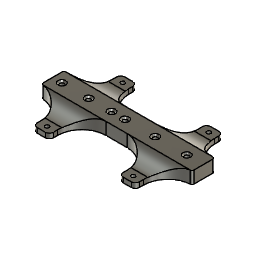
base (Autodesk Fusion 360 design; units mm, degrees)
Autodesk Fusion 360 part; units mm, degrees
sketch "Sketch1" plane through (0, 0, 0) normal (0, 0, 1) x (1, 0, 0)
  line L0 (0, 0) -> (186, 0)
  line L1 (186, 0) -> (186, 28)
  line L2 (186, 28) -> (0, 28)
  line L3 (0, 28) -> (0, 0)
  line L4 (0, 14) -> (186, 14) construction
  circle A0 centre (11.5, 14) radius 2.75
  circle A1 centre (44.5, 14) radius 2.75
  circle A2 centre (72.6667, 14) radius 2.75
  circle A3 centre (89.3333, 14) radius 2.75
  circle A4 centre (126.5, 14) radius 2.75
  circle A5 centre (165.5, 14) radius 2.75
  line L5 (13.8094, 10) -> (16.1188, 14)
  line L6 (16.1188, 14) -> (13.8094, 18)
  line L7 (13.8094, 18) -> (9.1906, 18)
  line L8 (9.1906, 18) -> (6.8812, 14)
  line L9 (6.8812, 14) -> (9.1906, 10)
  line L10 (9.1906, 10) -> (13.8094, 10)
  line L11 (46.8094, 10) -> (49.1188, 14)
  line L12 (49.1188, 14) -> (46.8094, 18)
  line L13 (46.8094, 18) -> (42.1906, 18)
  line L14 (42.1906, 18) -> (39.8812, 14)
  line L15 (39.8812, 14) -> (42.1906, 10)
  line L16 (42.1906, 10) -> (46.8094, 10)
  line L17 (74.9761, 10) -> (77.2855, 14)
  line L18 (77.2855, 14) -> (74.9761, 18)
  line L19 (74.9761, 18) -> (70.3573, 18)
  line L20 (70.3573, 18) -> (68.0479, 14)
  line L21 (68.0479, 14) -> (70.3573, 10)
  line L22 (70.3573, 10) -> (74.9761, 10)
  line L23 (91.6427, 10) -> (93.9521, 14)
  line L24 (93.9521, 14) -> (91.6427, 18)
  line L25 (91.6427, 18) -> (87.0239, 18)
  line L26 (87.0239, 18) -> (84.7145, 14)
  line L27 (84.7145, 14) -> (87.0239, 10)
  line L28 (87.0239, 10) -> (91.6427, 10)
  line L29 (128.8094, 10) -> (131.1188, 14)
  line L30 (131.1188, 14) -> (128.8094, 18)
  line L31 (128.8094, 18) -> (124.1906, 18)
  line L32 (124.1906, 18) -> (121.8812, 14)
  line L33 (121.8812, 14) -> (124.1906, 10)
  line L34 (124.1906, 10) -> (128.8094, 10)
  line L35 (167.8094, 10) -> (170.1188, 14)
  line L36 (170.1188, 14) -> (167.8094, 18)
  line L37 (167.8094, 18) -> (163.1906, 18)
  line L38 (163.1906, 18) -> (160.8812, 14)
  line L39 (160.8812, 14) -> (163.1906, 10)
  line L40 (163.1906, 10) -> (167.8094, 10)
  point P0 (11.5, 14)
  point P1 (44.5, 14)
  point P2 (72.6667, 14)
  point P3 (89.3333, 14)
  point P4 (126.5, 14)
  point P5 (165.5, 14)
  dimension "d1" = 186
  dimension "d2" = 28
  dimension "d3" = 5.5
  dimension "d4" = 11.5
  dimension "d5" = 5.5
  dimension "d6" = 44.5
  dimension "d7" = 5.5
  dimension "d8" = 5.5
  dimension "d9" = 5.5
  dimension "d10" = 5.5
  dimension "d11" = 72.6667
  dimension "d12" = 89.3333
  dimension "d13" = 20.5
  dimension "d14" = 126.5
  dimension "d18" = 4
  dimension "d19" = 4
  dimension "d20" = 4
  dimension "d21" = 4
  dimension "d22" = 4
  dimension "d23" = 4
  constraint horizontal L0
  constraint vertical L1
  constraint horizontal L2
  constraint vertical L3
  constraint coincident L0.start L3.end
  constraint midpoint L3 L4.start
  constraint midpoint L1 L4.end
  constraint coincident L4 P0
  constraint coincident L4 P1
  constraint coincident L4 P2
  constraint coincident L4 P3
  constraint coincident L4 P4
  constraint coincident L4 P5
  constraint coincident P0 A0.centre
  constraint coincident P1 A1.centre
  constraint coincident P2 A2.centre
  constraint coincident P3 A3.centre
  constraint coincident P4 A4.centre
  constraint coincident P5 A5.centre
  measures "d1" distance of L0.start L0.end
  measures "d2" distance of L0.start L2.end
  measures "d3" diameter of A0
  measures "d4" distance of L4.start P0
  measures "d5" diameter of A1
  measures "d6" distance of L3 P1
  measures "d7" diameter of A2
  measures "d8" diameter of A3
  measures "d9" diameter of A4
  measures "d10" diameter of A5
  measures "d11" distance of L3 P2
  measures "d12" distance of L3 P3 L0.start
  measures "d13" distance of L1 P5
  measures "d14" distance of L3 P4
  measures "d18" distance of P0 L10
  measures "d19" distance of P1 L16
  measures "d20" distance of P2 L22
  measures "d21" distance of P3 L28
  measures "d22" distance of P4 L34
  measures "d23" distance of P5 L40
extrude "Extrude1" add sketch "Sketch1" along normal blind 15 contours L0 L1 L2 L3 | L5 L6 L7 L8 L9 L10 | L11 L12 L13 L14 L15 L16 | L17 L18 L19 L20 L21 L22 | L23 L24 L25 L26 L27 L28 | L29 L30 L31 L32 L33 L34 | L35 L36 L37 L38 L39 L40
chamfer "Chamfer1" distance 2 angle 45 6 edges at (8.9361, 14.9944, 15) (41.9361, 14.9944, 15) (70.1028, 14.9944, 15) (86.7694, 14.9944, 15) (123.9361, 14.9944, 15) (162.9361, 14.9944, 15)
extrude "Extrude2" cut sketch "Sketch1" along normal blind 4 contours L5 L6 L7 L8 L9 L10 | L11 L12 L13 L14 L15 L16 | L17 L18 L19 L20 L21 L22 | L23 L24 L25 L26 L27 L28 | L29 L30 L31 L32 L33 L34 | L35 L36 L37 L38 L39 L40
sketch "Sketch2" plane through (0, 0, 0) normal (-1, 0, 0) x (0, -1, 0)
  line L0 (-28, 0) -> (0, 0)
  line L1 (0, 0) -> (0, 15)
  line L2 (0, 15) -> (-28, 15)
  line L3 (-28, 15) -> (-28, 0)
  line L4 (0, 0) -> (40, 0)
  line L5 (40, 0) -> (40, 6)
  line L6 (40, 6) -> (25, 6)
  arc A0 (0, 15) -> (25, 6) centre (25, 45.2222) ccw
  line L7 (0, 15) -> (-28, 0) construction
  line L8 (-28, 15) -> (0, 0) construction
  line L9 (-14, -17.2562) -> (-14, 34) construction
  line L10 (-28, 0) -> (-68, 0)
  arc A1 (-53, 6) -> (-28, 15) centre (-53, 45.2222) ccw
  line L11 (-68, 6) -> (-53, 6)
  line L12 (-68, 0) -> (-68, 6)
  dimension "d26" = 40
  constraint coincident L0.end L1.start
  constraint perpendicular L1 L4
  constraint perpendicular L4 L5
  constraint perpendicular L5 L6
  constraint tangent L6 A0
  constraint coincident L1.end L2.start
  constraint coincident L0.start L3.end
  constraint coincident L2.end L3.start
  constraint perpendicular L2 L9
  constraint symmetric L0.end L9 L0.start
  constraint symmetric L4.end L9 L10.end
  constraint symmetric L5.end L9 L11.start
  constraint symmetric L6.end L9 A1.start
  constraint symmetric L1.end L9 L2.end
  constraint symmetric A0 L9 A1
  measures "d26" distance of L0.end L4.end
extrude "Extrude3" add sketch "Sketch2" against normal blind 20 from surface at -30 contours L3 L10 A1 L11 L12 | L1 L4 L5 L6 A0
extrude "Extrude4" add sketch "Sketch2" along normal blind 20 from surface at -156 contours L3 L10 A1 L11 L12 | L1 L4 L5 L6 A0
fillet "Fillet1" radius 30 8 edges at (50, 0, 7.5) (30, 0, 7.5) (50, 28, 7.5) (136, 28, 7.5) (156, 28, 7.5) (156, 0, 7.5) (136, 0, 7.5) (30, 28, 7.5)
sketch "Sketch3" plane through (0, 0, 6) normal (0, 0, 1) x (-1, 0, 0)
  line L0 (-30, 30) -> (-30, 40)
  line L1 (-30, 40) -> (-50, 40)
  line L2 (-50, 40) -> (-50, 30)
  arc A0 (-50.4196, 25) -> (-50, 30) centre (-80, 30) ccw
  line L3 (-50.4196, 25) -> (-29.5804, 25)
  arc A1 (-30, 30) -> (-29.5804, 25) centre (0, 30) ccw
  line L4 (-156, 40) -> (-156, 30)
  arc A2 (-156.4196, 25) -> (-156, 30) centre (-186, 30) ccw
  line L5 (-156.4196, 25) -> (-135.5804, 25)
  arc A3 (-136, 30) -> (-135.5804, 25) centre (-106, 30) ccw
  line L6 (-136, 30) -> (-136, 40)
  line L7 (-136, 40) -> (-156, 40)
  line L8 (-156, -58) -> (-156, -68)
  line L9 (-156, -68) -> (-136, -68)
  line L10 (-136, -68) -> (-136, -58)
  arc A4 (-135.5804, -53) -> (-136, -58) centre (-106, -58) ccw
  line L11 (-135.5804, -53) -> (-156.4196, -53)
  arc A5 (-156, -58) -> (-156.4196, -53) centre (-186, -58) ccw
  line L12 (-30, -68) -> (-30, -58)
  arc A6 (-29.5804, -53) -> (-30, -58) centre (0, -58) ccw
  line L13 (-29.5804, -53) -> (-50.4196, -53)
  arc A7 (-50, -58) -> (-50.4196, -53) centre (-80, -58) ccw
  line L14 (-50, -58) -> (-50, -68)
  line L15 (-50, -68) -> (-30, -68)
  line L16 (-50.4196, 25) -> (-30, 40) construction
  line L17 (-29.5804, 25) -> (-50, 40) construction
  line L18 (-156, -68) -> (-135.5804, -53) construction
  line L19 (-136, -68) -> (-156.4196, -53) construction
  line L20 (-136, 40) -> (-156.4196, 25) construction
  line L21 (-135.5804, 25) -> (-156, 40) construction
  line L22 (-29.5804, -53) -> (-50, -68) construction
  line L23 (-30, -68) -> (-50.4196, -53) construction
  circle A8 centre (-40, -60.6541) radius 2.5
  circle A9 centre (-40, 32.6541) radius 2.5
  circle A10 centre (-146, 32.6541) radius 2.5
  circle A11 centre (-146, -60.6541) radius 2.5
  point P0 (-146, 32.6541)
  point P1 (-146, -60.6541)
  dimension "d35" = 5
  dimension "d36" = 5
  dimension "d37" = 5
  dimension "d38" = 5
  constraint coincident A0.start L3.start
  constraint coincident L0.end L1.start
  constraint coincident L3.end A1.end
  constraint coincident L1.end L2.start
  constraint coincident L8.end L9.start
  constraint coincident A4.start L11.start
  constraint coincident L9.end L10.start
  constraint coincident L11.end A5.end
  constraint coincident L6.end L7.start
  constraint coincident A2.start L5.start
  constraint coincident L5.end A3.end
  constraint coincident L4.start L7.end
  constraint coincident L21 P0
  constraint coincident L20 P0
  constraint coincident L18 P1
  constraint coincident L19 P1
  constraint coincident A6.start L13.start
  constraint coincident L14.end L15.start
  constraint coincident L12.start L15.end
  constraint coincident L13.end A7.end
  constraint coincident L22 A8.centre
  constraint coincident L23 A8.centre
  constraint coincident L17 A9.centre
  constraint coincident L16 A9.centre
  constraint coincident P0 A10.centre
  constraint coincident P1 A11.centre
  measures "d35" diameter of A8
  measures "d36" diameter of A9
  measures "d37" diameter of A10
  measures "d38" diameter of A11
extrude "Extrude5" cut sketch "Sketch3" against normal blind 6 contours A8 | A9 | A10 | A11
fillet "Fillet2" radius 2.5 4 edges at (186, 0, 7.5) (186, 28, 7.5) (0, 0, 7.5) (0, 28, 7.5)
fillet "Fillet3" radius 5 8 edges at (30, -40, 3) (50, -40, 3) (136, -40, 3) (156, -40, 3) (156, 68, 3) (136, 68, 3) (50, 68, 3) (30, 68, 3)
equation "d1 = 50 mm + 56 mm + 80 mm"
equation "d11 = 56 mm + ( 50 / 3 ) * 1 mm"
equation "d12 = 56 mm + ( 2 * 50 / 3 ) * 1 mm"
equation "d14 = 106 mm + 20.5 mm"
equation "d30 = -186 mm + 30.00 mm"
